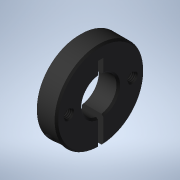
# Autodesk Inventor part: SCSWJ10-6_b
Saved by Autodesk Inventor 2021 (Build 250183000, 183)
## iProperties
Created: 2024-12-08
Part Number: SCSWJ10-6_b
Material: Generic
Catalog Web Link: www.cadenas.de
Description: SCSWJ, PSCSWJ, SSCSWJ_b-Set Collars - Slit 2 Hole/2 Tap - Compact Type - 2 Tap Type
Vendor: MISUMI
Document SubType Name: Modeling
Designer: psAdmin
Manufacturer: MISUMI
Mass: 2.12059 g
Surface Area: 17.2178 cm^2
Volume: 2.12059 cm^3
Density: 1 g/cm^3
Appearance: PSOLRGB-175-175-175
Category: PARTsolutions
Company: MISUMI
Title: SCSWJ10-6
Author: Cadenas PARTsolutions
Comments: Set Collars - Slit 2 Hole/2 Tap - Compact Type - 2 Tap Type
PSOL_IDENT_0: {$CADENAS_DATA/23d-libs/misumi/metric/03_set_collars/scswj/scswj_b.prj},183 {VTYP=3D},{NB=SCSWJ10-6_
PSOL_IDENT_1: b},{LINA=SCSWJ10-6},{NN=SCSWJ, PSCSWJ, SSCSWJ_b},{DATE=29.11.2024 04:05:21},{GEOMDATE=24.09.2021 04:
PSOL_IDENT_2: 03:07},{VERSION=},{LINEID=60},{WBVAR=MAT,ST},{WBNUMERIC=}  {NB=SCSWJ10-6_b},{LINA=SCSWJ10-6},{KT=DUM
PSOL_IDENT_3: MY},{PN=SCSWJ10-6},{TYPE=SCSWJ},{MAT=1045},{MATA='1045','S45C Equivalent','304','SUS304 Equivalent'}
PSOL_IDENT_4: ,{ST=BO},{ST0='BO','Black Oxide','ENP','Electroless Nickel Plating'},{AC=Hexagon Socket Head Set Scr
PSOL_IDENT_5: ew 1 Pc.},{D=10},{B=6},{D1=25},{M=M2.5},{THMD=2.5},{THDMIN=2.013},{DD=2.9},{R=2.45},{W=1.5},{X=8.0},
PSOL_IDENT_6: {Y=3},{Z=9.0},{P=18},{C=0.5},{L=10},{M1=M3},{THMD1=3},{THDMIN1=2.459}
NB: SCSWJ10-6_b
NN: SCSWJ, PSCSWJ, SSCSWJ_b
NT: Set Collars - Slit 2 Hole/2 Tap - Compact Type - 2 Tap Type
NBSYN: $PN._b
LINA: SCSWJ10-6
CATALOG: Misumi
PN: SCSWJ10-6
MAT: S45C Equivalent
ST: Black Oxide
AC: Hexagon Socket Head Set Screw 1 Pc.
D: 10
B: 6
D1: 25
M: M2.5
DD: 2.9
R: 2.45
W: 1.5
X: 8
Y: 3
Z: 9
P: 18
M1: M3
SUPPLIER: MISUMI
ARTICLENO: SCSWJ10-6_b
BOMINFO: SCSWJ10-6
CREATOR: CADENAS GmbH
Autodesk Inventor part; units mm, degrees
sketch "Sketch_1" plane through (0, 0, 0) normal (0, 0, 1) x (1, 0, 0)
  line L0 (3, 0) -> (-3, 0)
  line L1 (-3, 12) -> (-3, 5.5)
  line L2 (-3, 5.5) -> (-2.5, 5)
  line L3 (-2.5, 5) -> (2.5, 5)
  line L4 (2.5, 5) -> (3, 5.5)
  line L5 (3, 5.5) -> (3, 12)
  line L6 (3, 12) -> (2.5, 12.5)
  line L7 (2.5, 12.5) -> (-2.5, 12.5)
  line L8 (-2.5, 12.5) -> (-3, 12)
  constraints: 18 end point
revolve "Revolution1" add sketch "Sketch_1" angle 360 about axis through (3, 0, 0) along (1, 0, 0)
sketch "Sketch_2" plane through (0, 0, 0) normal (1, 0, 0) x (0, 1, 0)
  line L0 (-12.5, 0.75) -> (-12.5, -0.75)
  line L1 (-12.5, -0.75) -> (9, -0.75)
  line L2 (9, -0.75) -> (9, 0.75)
  line L3 (9, 0.75) -> (-12.5, 0.75)
  constraints: 8 end point
extrude "Extrusion1" cut sketch "Sketch_2" along normal mid plane 6
sketch "Sketch_3" plane through (0, 0, 0) normal (1, 0, 0) x (0, 1, 0)
  line L0 (-8, 12.5) -> (-8, 0)
  line L1 (-8, 0) -> (-9.45, 0)
  line L2 (-9.45, 0) -> (-9.45, 3)
  line L3 (-9.45, 3) -> (-10.45, 3)
  line L4 (-10.45, 3) -> (-10.45, 12.5)
  line L5 (-10.45, 12.5) -> (-8, 12.5)
  line L6 (-8, 12.5) -> (-8, 0)
  constraints: 14 end point
revolve "Revolution2" cut sketch "Sketch_3" angle 360 about axis through (0, -8, 12.5) along (0, 0, 1)
sketch "Sketch_4" plane through (0, 0, 0) normal (1, 0, 0) x (0, 1, 0)
  line L0 (-8, -12.75) -> (-8, -0.75)
  line L1 (-8, -0.75) -> (-6.75, -0.75)
  line L2 (-6.75, -0.75) -> (-6.9935, -0.9935)
  line L3 (-6.9935, -0.9935) -> (-6.9935, -12.75)
  line L4 (-6.9935, -12.75) -> (-8, -12.75)
  line L5 (-8, -12.75) -> (-8, -0.75)
  constraints: 12 end point
revolve "Revolution3" cut sketch "Sketch_4" angle 360 about axis through (0, -8, -12.75) along (0, 0, -1)
thread "Thread1" size "M2.5x0.45" class "6H" standard "ISO Metric profile" length 9.5273
sketch "Sketch_7" plane through (0, 0, -9) normal (0, 0, 1) x (1, 0, 0)
  line L0 (3, 0) -> (-3, 0)
  line L1 (-3, 0) -> (-3, 1.5)
  line L2 (-3, 1.5) -> (-2.7295, 1.2295)
  line L3 (-2.7295, 1.2295) -> (2.7295, 1.2295)
  line L4 (2.7295, 1.2295) -> (3, 1.5)
  line L5 (3, 1.5) -> (3, 0)
  line L6 (3, 0) -> (-3, 0)
  constraints: 14 end point
revolve "Revolution4" cut sketch "Sketch_7" angle 360 about axis through (3, 0, -9) along (1, 0, 0)
thread "Thread2" size "M3x0.5" class "6H" standard "ISO Metric profile" full length
sketch "Sketch_8" plane through (0, 0, 9) normal (0, 0, 1) x (1, 0, 0)
  line L0 (3, 0) -> (-3, 0)
  line L1 (-3, 0) -> (-3, 1.5)
  line L2 (-3, 1.5) -> (-2.7295, 1.2295)
  line L3 (-2.7295, 1.2295) -> (2.7295, 1.2295)
  line L4 (2.7295, 1.2295) -> (3, 1.5)
  line L5 (3, 1.5) -> (3, 0)
  line L6 (3, 0) -> (-3, 0)
  constraints: 14 end point
revolve "Revolution5" cut sketch "Sketch_8" angle 360 about axis through (3, 0, 9) along (1, 0, 0)
thread "Thread3" size "M3x0.5" class "6H" standard "ISO Metric profile" full length
ref_plane "body_screw_XY" through (0, -8, 3) normal (0, 0, 1) x (1, 0, 0)
ref_plane "body_screw_YZ" through (0, -8, 3) normal (1, 0, 0) x (0, 1, 0)
ref_plane "body_screw_ZX" through (0, -8, 3) normal (0, 1, 0) x (0, 0, 1)
body "Solid1"
